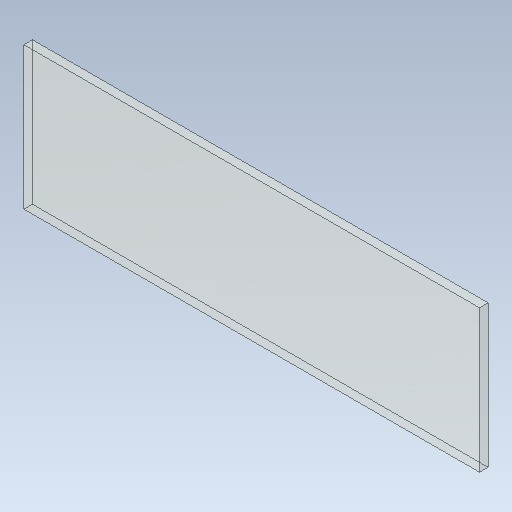
# Autodesk Inventor part: Vidrio
Saved by Autodesk Inventor 2020 (Build 240168000, 168)
## iProperties
Created: 2020-03-11
Part Number: Vidrio
Material: Vidrio
Document SubType Name: Modeling
Designer: joser
Density: 2.18 g/cm^3
Appearance: Claro
Author: joser
Autodesk Inventor part; units mm, degrees
ref_plane "YZ Plane" through (0, 0, 0) normal (1, 0, 0) x (0, 1, 0)
ref_plane "XZ Plane" through (0, 0, 0) normal (0, 1, 0) x (-1, 0, 0)
ref_plane "XY Plane" through (0, 0, 0) normal (0, 0, 1) x (1, 0, 0)
sketch "Boceto1" plane through (0, 0, 0) normal (0, 0, 1) x (1, 0, 0)
  line L0 (-80, -25) -> (80, -25)
  line L1 (80, -25) -> (80, 25)
  line L2 (80, 25) -> (-80, 25)
  line L3 (-80, 25) -> (-80, -25)
  line L4 (-80, -25) -> (80, 25) construction
  line L5 (80, -25) -> (-80, 25) construction
  point P0 (0, 0)
  dimension "d0" = 160
  dimension "d1" = 50
  constraints: 12 end point, 2 midpoint, 2 parallel, 1 horizontal, 1 perpendicular
  measures "d0" distance of L2.end L1.end
  measures "d1" distance of L1.end L0.end
extrude "Extrusión1" add sketch "Boceto1" along normal blind 3
